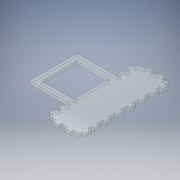
# Autodesk Inventor part: case_back
Saved by Autodesk Inventor 2019 (Build 230136000, 136)
## iProperties
Created: 2019-02-02
Part Number: case_back
Material: Acrylic, Clear
Document SubType Name: Modeling
Designer: suchanek
Density: 1.19 g/cm^3
Appearance: Transparent - Clear
Author: suchanek
Autodesk Inventor part; units mm, degrees
ref_plane "YZ Plane" through (0, 0, 0) normal (1, 0, 0) x (0, 1, 0)
ref_plane "XZ Plane" through (0, 0, 0) normal (0, 1, 0) x (-1, 0, 0)
ref_plane "XY Plane" through (0, 0, 0) normal (0, 0, 1) x (1, 0, 0)
sketch "Sketch1" plane through (0, 0, 0) normal (0, 1, 0) x (-1, 0, 0)
  line L0 (-30, 90) -> (30, 90)
  line L1 (30, 90) -> (30, -90)
  line L2 (30, -90) -> (-30, -90)
  line L3 (-30, -90) -> (-30, 90)
  line L4 (-30, 90) -> (30, -90) construction
  line L5 (30, 90) -> (-30, -90) construction
  line L6 (-30, 84) -> (-36, 84)
  line L7 (-36, 84) -> (-36, 72)
  line L8 (-36, 72) -> (-30, 72)
  line L9 (-30, 72) -> (-30, 84)
  line L10 (-36, 66) -> (-30, 66)
  line L11 (-30, 66) -> (-30, 54)
  line L12 (-30, 54) -> (-36, 54)
  line L13 (-36, 54) -> (-36, 66)
  line L14 (-30, 42) -> (-36, 42)
  line L15 (-36, 42) -> (-36, 30)
  line L16 (-36, 30) -> (-30, 30)
  line L17 (-30, 30) -> (-30, 42)
  line L18 (-30, 18) -> (-36, 18)
  line L19 (-36, 18) -> (-36, 6)
  line L20 (-36, 6) -> (-30, 6)
  line L21 (-30, 6) -> (-30, 18)
  line L22 (0, 0) -> (-5.6352, 0)
  line L23 (-5.6352, 0) -> (0, 0)
  line L24 (0, 0) -> (0, 8.7024)
  line L25 (-30, 90) -> (30, -90) construction
  line L26 (30, 84) -> (36, 84)
  line L27 (36, 84) -> (36, 72)
  line L28 (36, 72) -> (30, 72)
  line L29 (30, 72) -> (30, 84)
  line L30 (36, 66) -> (30, 66)
  line L31 (30, 66) -> (30, 54)
  line L32 (30, 54) -> (36, 54)
  line L33 (36, 54) -> (36, 66)
  line L34 (-30, -84) -> (-36, -84)
  line L35 (-36, -84) -> (-36, -72)
  line L36 (-36, -72) -> (-30, -72)
  line L37 (-30, -72) -> (-30, -84)
  line L38 (-36, -66) -> (-30, -66)
  line L39 (-30, -66) -> (-30, -54)
  line L40 (-30, -54) -> (-36, -54)
  line L41 (-36, -54) -> (-36, -66)
  line L42 (-30, -42) -> (-36, -42)
  line L43 (-36, -42) -> (-36, -30)
  line L44 (-36, -30) -> (-30, -30)
  line L45 (-30, -30) -> (-30, -42)
  line L46 (-30, -18) -> (-36, -18)
  line L47 (-36, -18) -> (-36, -6)
  line L48 (-36, -6) -> (-30, -6)
  line L49 (-30, -6) -> (-30, -18)
  line L50 (30, -84) -> (36, -84)
  line L51 (36, -84) -> (36, -72)
  line L52 (36, -72) -> (30, -72)
  line L53 (30, -72) -> (30, -84)
  line L54 (30, -54) -> (36, -54)
  line L55 (30, -66) -> (30, -54)
  line L56 (36, -66) -> (30, -66)
  line L57 (36, -54) -> (36, -66)
  line L58 (18, 90) -> (6, 90)
  line L59 (6, 90) -> (6, 96)
  line L60 (6, 96) -> (18, 96)
  line L61 (18, 96) -> (18, 90)
  line L62 (-18, 90) -> (-6, 90)
  line L63 (-6, 90) -> (-6, 96)
  line L64 (-6, 96) -> (-18, 96)
  line L65 (-18, 96) -> (-18, 90)
  line L66 (18, -90) -> (6, -90)
  line L67 (6, -90) -> (6, -96)
  line L68 (6, -96) -> (18, -96)
  line L69 (18, -96) -> (18, -90)
  line L70 (-18, -90) -> (-6, -90)
  line L71 (-6, -90) -> (-6, -96)
  line L72 (-6, -96) -> (-18, -96)
  line L73 (-18, -96) -> (-18, -90)
  line L74 (30, -48) -> (113, -48)
  line L75 (113, -48) -> (113, 48)
  line L76 (113, 48) -> (30, 48)
  line L77 (30, 48) -> (30, -48)
  line L78 (101, -36) -> (36, -36)
  line L79 (36, -36) -> (36, 36)
  line L80 (36, 36) -> (101, 36)
  line L81 (101, 36) -> (101, -36)
  circle A0 centre (33, 33) radius 1.5
  circle A1 centre (33, -33) radius 1.5
  point P0 (0, -8.7024)
  dimension "d0" = 60
  dimension "d1" = 180
  dimension "d2" = 6
  dimension "d3" = 6
  dimension "d4" = 12
  dimension "d5" = 12
  dimension "d6" = 12
  dimension "d7" = 12
  dimension "d8" = 12
  dimension "d9" = 6
  dimension "d10" = 12
  dimension "d17" = 6
  dimension "d19" = 6
  dimension "d20" = 6
  dimension "d21" = 6
  dimension "d22" = 12
  dimension "d23" = 12
  dimension "d24" = 12
  dimension "d25" = 6
  dimension "d26" = 65
  dimension "d27" = 12
  dimension "d28" = 3
  dimension "d29" = 3
  dimension "d30" = 3
  constraints: 164 end point, 46 symmetric about line, 17 equal length, 14 point on line, 9 horizontal, 8 perpendicular, 2 centre point, 2 midpoint, 1 vertical, 1 other
  measures "d0" distance of L1.end L2.end
  measures "d1" distance of L0.end L1.end
  measures "d2" distance of L19.end L20.end
  measures "d3" distance from line of L22.start L20
  measures "d4" distance of L18.end L19.end
  measures "d5" distance between parallel lines of L18 L16
  measures "d6" distance of L14.end L15.end
  measures "d7" distance between parallel lines of L12 L14
  measures "d8" distance of L12.end L10.start
  measures "d9" distance between parallel lines of L10 L8
  measures "d10" distance of L6.end L7.end
  measures "d17" distance of L58.end L59.end
  measures "d19" distance between parallel lines of L24 L59
  measures "d20" distance between parallel lines of L54 L74
  measures "d21" distance between parallel lines of L32 L76
  measures "d22" distance between parallel lines of L81 L75
  measures "d23" distance between parallel lines of L76 L80
  measures "d24" distance between parallel lines of L74 L78
  measures "d25" distance between parallel lines of L79 L77
  measures "d26" distance between parallel lines of L79 L81
  measures "d27" distance of L59.end L60.end
  measures "d28" diameter of A0
  measures "d29" distance from line of L79 A0.centre
  measures "d30" distance from line of L80 A0.centre
extrude "Extrusion1" add sketch "Sketch1" along normal blind 6
equation "\"d22\" = d23"
equation "\"d24\" = d23"
body "Solid1"
